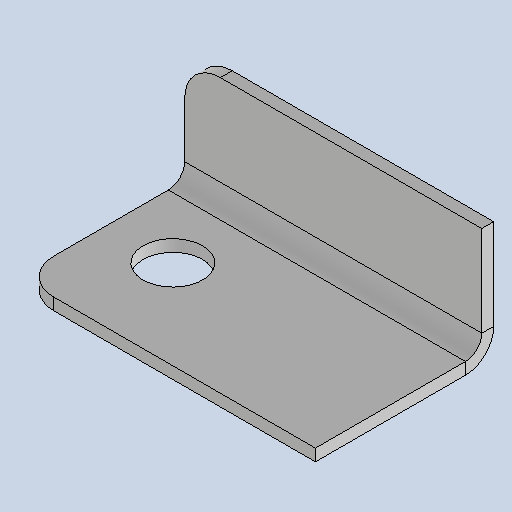
# Autodesk Inventor part: MSC 124 ROСKET PILLAR
Saved by Autodesk Inventor 2025 (Build 290162010, 162A)
## iProperties
Created: 2024-05-19
Part Number: MSC 124 ROСKET PILLAR
Material: Stainless Steel
Document SubType Name: Sheet Metal
Designer: admin
Stock Number: МОО 103 ракета нос
Mass: 14.9776 g
Surface Area: 48.5942 cm^2
Volume: 1.87221 cm^3
Density: 8 g/cm^3
Sheet Metal Rule: AISI304 2mm Die16
Sheet Metal Width: 50,000 mm
Sheet Metal Length: 46,202 mm
Sheet Metal Area: 2310,100 mm^2
Appearance: Default
Flat Pattern Width: 5 cm
Flat Pattern Length: 4.6202 cm
Flat Pattern Area: 23.101 cm^2
Author: admin
Autodesk Inventor part; units mm, degrees
ref_plane "YZ Plane" through (0, 0, 0) normal (1, 0, 0) x (0, 1, 0)
ref_plane "XZ Plane" through (0, 0, 0) normal (0, 1, 0) x (-1, 0, 0)
ref_plane "XY Plane" through (0, 0, 0) normal (0, 0, 1) x (1, 0, 0)
sketch "Sketch2" plane through (0, 0, 0) normal (0, 0, 1) x (1, 0, 0)
  line L0 (0, 0) -> (0, 30)
  line L1 (0, 30) -> (-50, 30)
  line L2 (-50, 30) -> (-50, 0)
  line L3 (-50, 0) -> (0, 0)
  dimension "d10" = 30
  dimension "d30" = 50
  measures "d10" distance of L0.start L0.end
  measures "d30" distance of L0.end L1.end
extrude "Plate1" add sketch "Sketch2" along normal blind 2
sketch "Sketch3" plane through (-50, 28, 0) normal (0, 1, 0) x (-1, 0, 0)
  line L0 (-50, 0) -> (0, 0)
  line L1 (0, 0) -> (0, 20)
  line L2 (0, 20) -> (-50, 20)
  line L3 (-50, 20) -> (-50, 0)
  constraints: 6 end point, 1 horizontal, 1 perpendicular, 1 vertical
edge flange "Flange1" height 20 angle 90 thickness 2 bend radius 2.75 thickness toward (0, 1, 0) relief round relief width 2 relief depth 1 edges at (-25, 30, 2) wall of the first edge with corners at (0, 28, 0) (-50, 28, 0) (-50, 28, 20) (0, 28, 20)
bend "Bend1"
corner "Corner1"
fillet "Corner Round1" radius 6 2 edges at (-50, 0, 1) (-50, 29, 20)
sketch "Sketch4" plane through (0, 0, 0) normal (0, 0, -1) x (-1, 0, 0)
  circle A0 centre (39, 15) radius 5
  line L0 (44, 0) -> (0, 0) projected
  dimension "d25" = 10
  dimension "d26" = 15
  dimension "d27" = 5
  constraints: 1 centre point
  measures "d25" diameter of A0
  measures "d26" distance from line of L0 A0.centre
  measures "d27" horizontal distance of L0.start A0.centre
extrude "Cut1" cut sketch "Sketch4" against normal blind 2
equation "\"d28\" = Thickness"
equation "\"d7\" = Thickness"
equation "\"d14\" = BendReliefWidth"
equation "\"d15\" = BendReliefDepth"
equation "\"d16\" = MinimumRemnant"
equation "\"d17\" = TransitionRadius"
equation "\"d20\" = BendRadius"
equation "\"d21\" = CornerReliefSize"
equation "\"d22\" = GapSize"
equation "\"d23\" = JacobiRadiusSize"
equation "\"BendReliefWidth\" = Thickness"
equation "\"BendReliefDepth\" = 0.5 * Thickness"
equation "\"CornerReliefSize\" = 4 * Thickness"
equation "\"MinimumRemnant\" = 2 * Thickness"
equation "\"TransitionRadius\" = BendRadius"
equation "\"JacobiRadiusSize\" = BendRadius"
equation "\"GapSize\" = Thickness"
equation "\"Thickness\" = 2"
equation "\"BendRadius\" = 2.75"
body "Solid2"
